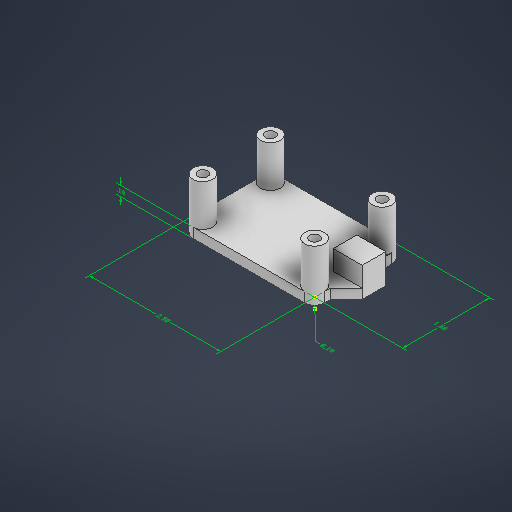
# Autodesk Inventor part: MotorBot
Saved by Autodesk Inventor 2026 (Build 300175000, 175)
## iProperties
Created: 2025-04-10
Part Number: MotorBot
Material: Generic
Document SubType Name: Modeling
Designer: jjgen
Density: 1 g/cm^3
Appearance: Default
Author: jjgen
## iProperties of the stored document MotorBot_3DPrint.ipt
Created: 2025-04-17
Part Number: MotorBot_3DPrint
Material: Generic
Document SubType Name: Modeling
Designer: sdcel
Density: 1 g/cm^3
Appearance: Default
Author: sdcel
Autodesk Inventor part; units mm, degrees
ref_plane "YZ Plane" through (0, 0, 0) normal (1, 0, 0) x (0, 1, 0)
ref_plane "XZ Plane" through (0, 0, 0) normal (0, 1, 0) x (-1, 0, 0)
ref_plane "XY Plane" through (0, 0, 0) normal (0, 0, 1) x (1, 0, 0)
sketch "Sketch1" plane through (0, 0, 0) normal (0, 1, 0) x (-1, 0, 0)
  point P0 (0, 0)
sketch "Sketch2" plane through (0, 0, 0) normal (0, 1, 0) x (-1, 0, 0)
  line L0 (0, -4.7625) -> (0, -37.4015)
  line L1 (4.7625, -42.164) -> (58.7375, -42.164)
  line L2 (63.5, -37.4015) -> (63.5, -4.7625)
  line L3 (58.7375, 0) -> (4.7625, 0)
  arc A0 (4.7625, 0) -> (0, -4.7625) centre (4.7625, -4.7625) ccw
  circle A1 centre (4.7625, -4.7625) radius 4.7625
  circle A2 centre (4.7625, -4.7625) radius 2.3813
  arc A3 (0, -37.4015) -> (4.7625, -42.164) centre (4.7625, -37.4015) ccw
  arc A4 (58.7375, -42.164) -> (63.5, -37.4015) centre (58.7375, -37.4015) ccw
  arc A5 (63.5, -4.7625) -> (58.7375, 0) centre (58.7375, -4.7625) ccw
  circle A6 centre (58.7375, -4.7625) radius 4.7625
  circle A7 centre (58.7375, -37.4015) radius 4.7625
  circle A8 centre (58.7375, -4.7625) radius 2.3813
  circle A9 centre (58.7375, -37.4015) radius 2.3813
  point P0 (0, 0)
  point P1 (0, -42.164)
  point P2 (63.5, -42.164)
  point P3 (4.7625, 0)
  point P4 (4.7625, 0)
  dimension "d0" = 42.164
  dimension "d1" = 63.5
  dimension "d2" = 4.7625
  dimension "d3" = 4.7625
  dimension "d4" = 4.7625
  dimension "d5" = 4.7625
  dimension "d6" = 4.7625
  constraints: 9 centre point, 8 end point, 8 point on circle, 8 tangent, 6 coincident, 6 point on line, 3 perpendicular, 2 equal radius, 1 vertical, 3 other
  measures "d0" distance of point (0, 0) point (0, -42.164)
  measures "d1" distance of point (0, -42.164) point (63.5, -42.164)
  measures "d2" radius of A0
  measures "d3" diameter of A2
  measures "d4" radius of A3
  measures "d5" diameter of A8
  measures "d6" diameter of A9
extrude "Extrusion1" add sketch "Sketch2" along normal blind 9.525 contours A0 A1 | A5 A6 | A7 A4
extrude "Extrusion2" add sketch "Sketch2" along normal blind 4.7625 contours A1 L3 A6 L2 A7 L1 A3 L0
sketch "Sketch3" plane through (0, 4.7625, 0) normal (0, 1, 0) x (1, 0, 0)
  circle A0 centre (-4.7625, 4.7625) radius 2.3813 projected
  line L0 (-4.7625, 4.7625) -> (-1.3949, 1.3949)
  circle A1 centre (-4.7625, 4.7625) radius 4.7625 projected
  line L1 (-4.7625, 4.7625) -> (0, 4.7625) construction
  circle A2 centre (-4.7625, 4.7625) radius 4.7625
  circle A3 centre (-4.7625, 4.7625) radius 2.3813
  circle A4 centre (-58.7375, 4.7625) radius 4.7625 projected
  circle A5 centre (-58.7375, 4.7625) radius 4.7625
  circle A6 centre (-58.7375, 4.7625) radius 2.3813
  circle A7 centre (-58.7375, 37.4015) radius 2.3813 projected
  circle A8 centre (-58.7375, 37.4015) radius 4.7625
  circle A9 centre (-58.7375, 37.4015) radius 2.3813 projected
  circle A10 centre (-58.7375, 37.4015) radius 2.3813
  point P0 (0, 0)
  dimension "d22" = 45
  constraints: 6 centre point, 6 coincident, 4 end point, 1 concentric, 1 equal length, 1 horizontal, 3 other
  measures "d22" angle of L0 L1
extrude "Extrusion3" add sketch "Sketch3" along normal blind 20.0025
sketch "Sketch4" plane through (0, 4.7625, 0) normal (0, 1, 0) x (1, 0, 0)
  line L0 (0, 4.7625) -> (0, 37.4015) projected
  line L1 (0, 21.082) -> (0, 26.797)
  line L2 (0, 26.797) -> (0, 21.082)
  line L3 (0, 21.082) -> (0, 15.367)
  line L4 (0, 15.367) -> (7.62, 15.367)
  line L5 (7.62, 15.367) -> (7.62, 26.797)
  line L6 (7.62, 26.797) -> (0, 26.797)
  line L7 (7.62, 26.797) -> (0, 34.417)
  line L8 (7.62, 26.797) -> (18.3963, 26.797) construction
  line L9 (7.62, 15.367) -> (0, 7.747)
  line L10 (7.62, 15.367) -> (18.3963, 15.367) construction
  point P0 (0, 0)
  dimension "d25" = 5.715
  dimension "d26" = 5.715
  dimension "d27" = 7.62
  dimension "d28" = 135
  dimension "d29" = 135
  constraints: 20 end point, 4 point on line, 3 perpendicular, 2 equal length, 2 horizontal, 1 collinear, 1 midpoint
  measures "d25" distance of L1.start L1.end
  measures "d26" distance of L1.start L3.end
  measures "d27" distance of L3.end L4.end
  measures "d28" angle of L8 L7
  measures "d29" angle of L9 L10
extrude "Extrusion4" add sketch "Sketch4" against normal blind 4.7625
sketch "Sketch5" plane through (0, 4.7625, 0) normal (0, 1, 0) x (1, 0, 0)
  line L0 (7.62, 26.797) -> (7.62, 15.367) projected
  line L1 (7.62, 15.367) -> (-6.35, 15.367)
  line L2 (-6.35, 15.367) -> (-6.35, 26.797)
  line L3 (-6.35, 26.797) -> (7.62, 26.797)
  line L4 (0, 7.747) -> (7.62, 15.367) projected
  line L5 (7.62, 15.367) -> (7.62, 26.797) projected
  line L6 (7.62, 15.367) -> (7.62, 26.797)
  point P0 (0, 0)
  dimension "d32" = 13.97
  constraints: 8 end point, 2 perpendicular, 1 collinear, 1 horizontal
  measures "d32" distance of L0.end L1.end
sketch "Sketch6" plane through (0, 4.7625, 0) normal (0, 1, 0) x (1, 0, 0)
  point P0 (0, 0)
extrude "Extrusion5" add sketch "Sketch5" along normal blind 9.525
sketch "Sketch7" plane through (7.62, 0, -15.367) normal (1, 0, 0) x (0, 0, -1)
  line L0 (0, 4.7625) -> (11.43, 4.7625) projected
  line L1 (5.715, 4.7625) -> (5.715, 17.145)
  circle A0 centre (5.715, 17.145) radius 5.715
  point P0 (-15.367, 0)
  dimension "d35" = 12.3825
  dimension "d36" = 11.43
  constraints: 2 end point, 1 centre point, 1 coincident, 1 midpoint, 1 vertical
  measures "d35" distance of L1.start L1.end
  measures "d36" diameter of A0
extrude "Extrusion6" cut sketch "Sketch7" against normal blind 9.9441
sketch "Sketch8" plane through (0, 4.7625, 0) normal (0, 1, 0) x (1, 0, 0)
  line L0 (-58.7375, 0) -> (-4.7625, 0) projected
  line L1 (-31.75, 0) -> (-31.75, 42.164)
  line L2 (-4.7625, 42.164) -> (-58.7375, 42.164) projected
  circle A0 centre (-31.75, 21.082) radius 2.3812
  point P0 (0, 0)
  dimension "d39" = 4.7625
  constraints: 3 midpoint, 2 end point, 1 centre point
  measures "d39" diameter of A0
extrude "Extrusion7" cut sketch "Sketch8" against normal blind 9.9441
sketch "Sketch9" plane through (0, 0, 0) normal (0, -1, 0) x (1, 0, 0)
  arc A0 (-4.7625, -42.164) -> (0, -37.4015) centre (-4.7625, -37.4015) ccw projected
  circle A1 centre (-4.7625, -37.4015) radius 2.3813
  circle A2 centre (-4.7625, -4.7625) radius 2.3813 projected
  point P0 (0, 0)
  constraints: 1 centre point, 1 coincident, 1 equal radius
extrude "Extrusion8" cut sketch "Sketch9" against normal up to surface (4.7625 mm away) contours A1
sketch "Sketch10" plane through (0, 4.7625, 0) normal (0, 1, 0) x (1, 0, 0)
  circle A0 centre (-4.7625, 37.4015) radius 2.3813 projected
  circle A1 centre (-4.7625, 37.4015) radius 4.7625
  point P0 (0, 0)
  constraints: 1 centre point, 1 coincident
extrude "Extrusion9" add sketch "Sketch10" along normal up to surface (20.0025 mm away)
sketch "Sketch11" plane through (0, 4.7625, 0) normal (0, 1, 0) x (1, 0, 0)
  circle A0 centre (-31.75, 21.082) radius 2.3812 projected
  circle A1 centre (-31.75, 21.082) radius 2.3812
  point P0 (0, 0)
  constraints: 1 centre point, 1 coincident
extrude "Extrusion10" add sketch "Sketch11" against normal up to surface (4.7625 mm away)
sketch "Sketch12" plane through (-2.3241, 0, -15.367) normal (1, 0, 0) x (0, 0, -1)
  arc A0 (0.7657, 14.2875) -> (10.6643, 14.2875) centre (5.715, 17.145) ccw projected
  circle A1 centre (5.715, 17.145) radius 5.715
  line L0 (0.7657, 14.2875) -> (10.6643, 14.2875)
  line L1 (11.43, 14.2875) -> (0, 14.2875) projected
  point P0 (-15.367, 0)
  constraints: 2 end point, 1 centre point, 1 coincident, 1 collinear
extrude "Extrusion11" add sketch "Sketch12" along normal up to surface (9.9441 mm away) contours L0 A0
body "Solid1"
